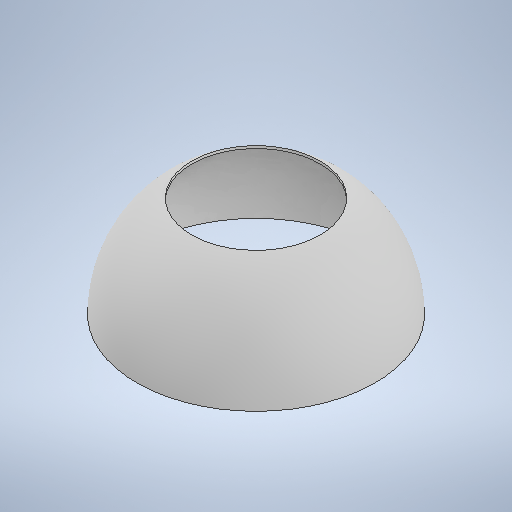
# Autodesk Inventor part: Ball
Saved by Autodesk Inventor 2025 (Build 290162000, 162)
## iProperties
Created: 2024-11-17
Part Number: Ball
Material: Generic
Document SubType Name: Modeling
Designer: ethan
Density: 1 g/cm^3
Appearance: Default
Author: ethan
Autodesk Inventor part; units mm, degrees
ref_plane "YZ Plane" through (0, 0, 0) normal (1, 0, 0) x (0, 1, 0)
ref_plane "XZ Plane" through (0, 0, 0) normal (0, 1, 0) x (-1, 0, 0)
ref_plane "XY Plane" through (0, 0, 0) normal (0, 0, 1) x (1, 0, 0)
sketch "Sketch1" plane through (0, 0, 0) normal (0, 1, 0) x (-1, 0, 0)
  line L0 (0, 0) -> (25, 0)
  line L1 (25, 0) -> (25, -25)
  line L2 (25, -25) -> (0, -25)
  line L3 (0, -25) -> (0, 0)
  circle A0 centre (12.5, -12.5) radius 17.6777
  circle A1 centre (12.5, -12.5) radius 21.86
  dimension "d0" = 25
  dimension "d1" = 25
  dimension "d2" = 43.72
  constraints: 8 end point, 2 parallel, 1 centre point, 1 coincident, 1 horizontal, 1 perpendicular, 3 other
  measures "d0" distance of L1.end L2.end
  measures "d1" distance of L0.end L1.end
  measures "d2" diameter of A1
extrude "Extrusion1" add sketch "Sketch1" along normal blind 1 contours L0 L1 L2 L3
ref_plane "Work Plane2" through (0, 0, 0) normal (-0.7071068, 0, 0.7071068) x (0, 1, 0)
sketch "Sketch3" plane through (0, 0, 0) normal (-0.7071068, 0, 0.7071068) x (0, 1, 0)
  line L0 (1, 0) -> (1, 17.6777) projected
  line L1 (1, 17.6777) -> (1, 35.3553) projected
  line L2 (1, 17.6777) -> (7.5, 17.6777) construction
  arc A0 (1, 0) -> (1, 35.3553) centre (-19.7885, 17.6777) ccw construction
  circle A1 centre (-19.7885, 17.6777) radius 27.375 construction
  circle A2 centre (-19.7885, 17.6777) radius 27.375
  circle A3 centre (-19.7885, 17.6777) radius 27.875
  line L3 (7.5, 17.6777) -> (8.0865, 17.6777)
  line L4 (-19.7885, 45.0527) -> (-19.7885, 45.5527)
  line L5 (-19.7885, 17.6777) -> (-5.3263, 17.6777)
  line L6 (-19.7885, 17.6777) -> (-19.7885, 45.0527)
  point P0 (0, 0)
  point P1 (7.5865, 17.6777)
  dimension "d10" = 6.5
  dimension "d11" = 54.75
  dimension "d12" = 55.75
  constraints: 10 end point, 7 point on circle, 4 centre point, 3 coincident, 3 horizontal, 1 concentric, 1 perpendicular, 1 vertical
  measures "d10" distance of L0.end L2.end
  measures "d11" diameter of A1
  measures "d12" diameter of A3
revolve "Revolution1" add sketch "Sketch3" angle 360 about axis through (-12.5, -19.7885, -12.5) along (0, 1, 0) picked at (-9.7302, 43.3292) contours A2 L4 A3 L3
ref_plane "Work Plane3" through (0, 1, 0) normal (0, -1, 0) x (1, 0, 0)
sketch "Sketch5" plane through (0, 0, 0) normal (0, -1, 0) x (1, 0, 0)
  line L0 (0, -25) -> (-25, -25) construction
  line L1 (0, 0) -> (0, -25) construction
  line L2 (-25, 0) -> (0, 0) construction
  line L3 (-25, -25) -> (-25, 0) construction
  line L4 (-12.5, 0) -> (-12.5, -12.5) construction
  circle A0 centre (-12.5, -12.5) radius 15
  dimension "d33" = 12.5
  dimension "d34" = 30
  constraints: 2 end point, 1 centre point, 1 coincident, 1 midpoint, 1 vertical
  measures "d33" distance of L4.start L4.end
  measures "d34" diameter of A0
extrude "Extrusion3" cut sketch "Sketch5" against normal blind 10
sketch "Sketch6" plane through (0, 0, 0) normal (0, -1, 0) x (1, 0, 0)
  arc A0 (-25, -20.7916) -> (-20.7916, -25) centre (-12.5, -12.5) ccw projected
  line L0 (0, -25) -> (-4.2084, -25) projected
  line L1 (0, 0) -> (0, -4.2084) projected
  line L2 (-25, 0) -> (-20.7916, 0) projected
  line L3 (-25, -25) -> (-25, -20.7916) projected
  line L4 (-20.7916, -25) -> (-25, -25) projected
  arc A1 (-4.2084, -25) -> (0, -20.7916) centre (-12.5, -12.5) ccw projected
  line L5 (0, -20.7916) -> (0, -25) projected
  arc A2 (0, -4.2084) -> (-4.2084, 0) centre (-12.5, -12.5) ccw projected
  line L6 (-4.2084, 0) -> (0, 0) projected
  arc A3 (-20.7916, 0) -> (-25, -4.2084) centre (-12.5, -12.5) ccw projected
  line L7 (-25, -4.2084) -> (-25, 0) projected
extrude "Extrusion4" cut sketch "Sketch6" against normal blind 1
body "Solid1"
